Autodesk Fusion 360 part; units mm, degrees
(part 3 of 3)
  line L37 (-24.3625, -11.1222) -> (-23.4964, -10.7273)
  arc A75 (-22.1886, -11.187) -> (-23.4964, -10.7273) centre (-23.0815, -11.6372) ccw
  arc A76 (-22.1886, -11.187) -> (-21.5014, -12.4568) centre (0, 0) ccw
  circle A77 centre (0, 15) radius 2.5
  circle A78 centre (-10.6066, 10.6066) radius 2.5
  circle A79 centre (-15, 0) radius 2.5
  circle A80 centre (-10.6066, -10.6066) radius 2.5
  circle A81 centre (0, -15) radius 2.5
  circle A82 centre (10.6066, -10.6066) radius 2.5
  circle A83 centre (15, 0) radius 2.5
  circle A84 centre (10.6066, 10.6066) radius 2.5
  dimension "d29" = 5
  dimension "d30" = 15
  dimension "d32" = 360
  measures "d29" diameter of A77
  measures "d30" distance of A77.centre A0.centre
component "Spur Gear (19 teeth)" placed x (1, 0, 0) y (0, 1, 0) z (0, 0, 1) at (0, 0, 0)
